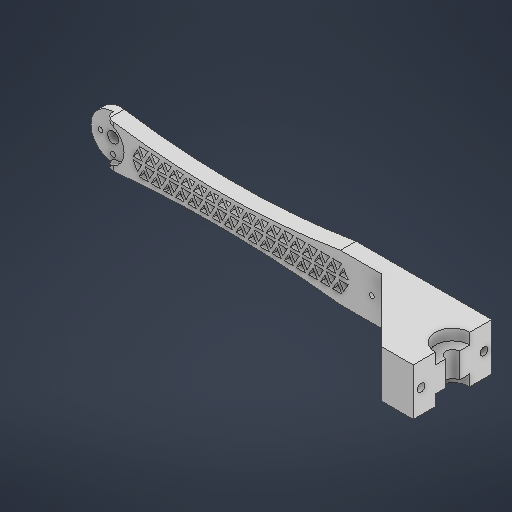
# Autodesk Inventor part: PeçaCerta
Saved by Autodesk Inventor 2026 (Build 300175050, 175E)
## iProperties
Created: 2025-03-07
Part Number: PeçaCerta
Material: Genérico
Document SubType Name: Modeling
Designer: Ian
Density: 1 g/cm^3
Appearance: Padrão
Mass: 116.041 g
Surface Area: 272.444 cm^2
Volume: 116.041 cm^3
Author: Ian
Autodesk Inventor part; units mm, degrees
ref_plane "YZ Plane" through (0, 0, 0) normal (1, 0, 0) x (0, 1, 0)
ref_plane "XZ Plane" through (0, 0, 0) normal (0, 1, 0) x (-1, 0, 0)
ref_plane "XY Plane" through (0, 0, 0) normal (0, 0, 1) x (1, 0, 0)
sketch "Esboço1" plane through (0, 0, 0) normal (0, 0, 1) x (1, 0, 0)
  circle A0 centre (-0.0013, -9.4999) radius 1.5997
  circle A1 centre (8, 0) radius 1.6001
  circle A2 centre (-8, 0) radius 1.5997
  circle A3 centre (0, 0) radius 3.5
  circle A4 centre (-0.0004, 9.5) radius 1.6001
  line L0 (0, 9.8096) -> (0, -11.1096)
  line L1 (-6.3022, 0) -> (16.3218, 0)
  line L2 (-14.0997, 15) -> (235.9003, 15)
  line L3 (235.9003, 15) -> (235.9003, -15)
  line L4 (235.9003, -15) -> (-14.0997, -15)
  line L5 (-14.0997, -15) -> (-14.0997, 15)
  point P0 (-14.0997, 0)
  dimension "d13" = 18.9999
  dimension "d37" = 9.2196
  dimension "d38" = 9.2197
  dimension "d39" = 9.2198
  dimension "d42" = 7
  dimension "d43" = 16
  dimension "d45" = 9.2207
  dimension "d46" = 4.5
  dimension "d47" = 250
  dimension "d48" = 30
  dimension "d49" = 0
  constraints: 12 end point, 5 centre point, 3 horizontal, 2 equal radius, 2 point on line, 2 vertical, 1 coincident, 1 midpoint, 1 parallel, 1 perpendicular
  measures "d13" distance of A4.centre A0.centre
  measures "d42" diameter of A3
  measures "d43" distance of A1.centre A2.centre
  measures "d46" distance edge to line of A2 L5
  measures "d47" distance of L2.start L2.end
  measures "d48" distance of L4.end L2.start
  measures "d49" vertical distance of A3.centre point (-14.1, 0)
extrude "Extrusão7" add sketch "Esboço1" along normal blind 10
sketch "Esboço13" plane through (0, 0, 0) normal (0, 0, -1) x (-1, 0, 0)
  line L0 (14.0997, -15) -> (-235.9003, -15) projected
  circle A0 centre (8, 0) radius 1.5997 projected
  circle A1 centre (0, 0) radius 3.5 projected
  circle A2 centre (0.0013, -9.4999) radius 1.5997 projected
  circle A3 centre (-8, 0) radius 1.6001 projected
  circle A4 centre (0.0004, 9.5) radius 1.6001 projected
  circle A5 centre (0, 0) radius 3.5
  circle A6 centre (-8, 0) radius 1.6001
  circle A7 centre (0.0013, -9.4999) radius 1.5997
  circle A8 centre (8, 0) radius 1.5997
  circle A9 centre (0.0004, 9.5) radius 1.6001
  line L1 (14.0997, 15) -> (14.0997, -15) projected
  line L2 (-14.0997, 15) -> (14.0997, 15)
  line L3 (14.0997, 15) -> (14.0997, -15)
  line L4 (14.0997, -15) -> (-14.0997, -15)
  line L5 (-14.0997, -15) -> (-14.0997, 15)
  line L6 (-14.0997, 15) -> (14.0997, -15) construction
  line L7 (14.0997, 15) -> (-14.0997, -15) construction
  circle A10 centre (0, 0) radius 14.0997
  point P0 (0, 0)
  point P1 (-15, -15)
  point P2 (-14.0997, -15)
  constraints: 12 end point, 6 centre point, 6 coincident, 5 concentric, 2 midpoint, 2 parallel, 1 horizontal, 1 perpendicular, 1 point on line
extrude "Extrusão11" add sketch "Esboço13" along normal blind 4
sketch "Esboço18" plane through (0, 0, 10) normal (0, 0, 1) x (1, 0, 0)
  line L0 (14.0997, -15) -> (235.9003, -15) projected
  line L1 (235.9003, 15) -> (14.0997, 15) projected
  line L2 (235.9003, -15) -> (175.9003, -15)
  line L3 (175.9003, -15) -> (175.9003, 15)
  line L4 (175.9003, 15) -> (235.9003, 15)
  line L5 (235.9003, 15) -> (235.9003, -15)
  point P0 (0, 0)
  dimension "d81" = 60
  constraints: 8 end point, 2 parallel, 1 horizontal, 1 perpendicular, 1 point on line
  measures "d81" distance of L3.end L4.end
extrude "Extrusão14" add sketch "Esboço18" along normal blind 40
sketch "Esboço19" plane through (14.0997, -15, 0) normal (0, -1, 0) x (1, 0, 0)
  line L0 (-28.1994, 10) -> (161.8006, 10) projected
  line L1 (161.8006, 10) -> (201.8006, 50)
  line L2 (221.8006, 50) -> (161.8006, 50) projected
  line L3 (201.8006, 50) -> (161.8006, 50)
  line L4 (161.8006, 10) -> (161.8006, 50)
  point P0 (-14.0997, 0)
  point P1 (0.4142, 10)
  point P2 (5, 10)
  point P3 (5, 10)
  point P4 (5.4142, 10)
  dimension "d84" = 45
  constraints: 6 end point, 1 collinear, 1 perpendicular, 1 point on line
  measures "d84" angle of L2 L1
extrude "Extrusão15" cut sketch "Esboço19" against normal through all
sketch "Esboço20" plane through (14.0997, -15, 0) normal (0, -1, 0) x (1, 0, 0)
  line L0 (161.8006, 10) -> (221.8006, 10)
  line L1 (221.8006, 0) -> (221.8006, 50) projected
  line L2 (221.8006, 50) -> (201.8006, 50) projected
  line L3 (201.8006, 50) -> (191.8006, 10)
  circle A0 centre (221.8006, 25) radius 10.975
  point P0 (-14.0997, 0)
  point P1 (221.8006, 35.975)
  point P2 (221.8006, 14.025)
  dimension "d87" = 21.95
  constraints: 4 end point, 2 midpoint, 1 centre point, 1 horizontal, 1 point on line
  measures "d87" diameter of A0
extrude "Extrusão16" cut sketch "Esboço20" against normal blind 7 contours A0 L1 picked at (218.1689, 24.559)
sketch "Esboço21" plane through (14.0997, -8, 0) normal (0, -1, 0) x (1, 0, 0)
  line L0 (221.8006, 35.975) -> (221.8006, 14.025) projected
  arc A0 (221.8006, 35.975) -> (221.8006, 14.025) centre (221.8006, 25) ccw projected
  circle A1 centre (221.8006, 25) radius 4.25
  point P0 (-14.0997, 0)
  point P1 (221.8006, 20.75)
  point P2 (221.8006, 29.25)
  dimension "d90" = 8.5
  constraints: 1 centre point, 1 coincident
  measures "d90" diameter of A1
extrude "Extrusão17" cut sketch "Esboço21" against normal through all contours L0 A1 picked at (220.3943, 24.8292)
sketch "Esboço22" plane through (14.0997, 15, 0) normal (0, 1, 0) x (1, 0, 0)
  arc A0 (221.8006, -20.75) -> (221.8006, -29.25) centre (221.8006, -25) ccw projected
  circle A1 centre (221.8006, -25) radius 10.975
  point P0 (-14.0997, 0)
  dimension "d93" = 21.95
  dimension "d173" = 4.25
  constraints: 1 centre point, 1 coincident
  measures "d93" diameter of A1
  measures "d173" radius of A0
extrude "Extrusão18" cut sketch "Esboço22" against normal blind 7
sketch "Esboço23" plane through (235.9003, -15, 0) normal (1, 0, 0) x (0, 0, -1)
  line L0 (-14.025, 30) -> (-14.025, 23) projected
  line L1 (-14.025, 7) -> (-14.025, 0) projected
  line L2 (-10, 0) -> (-10, 30) projected
  line L3 (-10, 30) -> (0, 30)
  circle A0 centre (-5, 15) radius 2.5
  line L4 (0, 15) -> (-50, 15)
  line L5 (-50, 30) -> (-50, 0) projected
  line L6 (-20.75, 23) -> (-20.75, 7) projected
  circle A1 centre (-45, 15) radius 2.5
  line L7 (-29.25, 7) -> (-29.25, 23) projected
  dimension "d96" = 5
  dimension "d174" = 15.75
  dimension "d175" = 5
  dimension "d177" = 15.75
  constraints: 4 end point, 2 centre point, 1 horizontal, 1 midpoint, 1 point on line
  measures "d96" diameter of A0
  measures "d174" distance from line of L6 A0.centre
  measures "d175" diameter of A1
  measures "d177" distance from line of L7 A1.centre
extrude "Extrusão19" cut sketch "Esboço23" against normal blind 50
sketch "Esboço24" plane through (0, 0, 0) normal (0, 0, -1) x (-1, 0, 0)
  line L0 (-235.9003, -2.5) -> (-235.9003, 2.5) projected
  line L1 (-175.9003, -15) -> (-175.9003, 15) projected
  line L2 (-183.4003, -12.5) -> (-208.4003, -12.5)
  line L3 (-208.4003, -12.5) -> (-208.4003, 12.5)
  line L4 (-208.4003, 12.5) -> (-183.4003, 12.5)
  line L5 (-183.4003, 12.5) -> (-183.4003, -12.5)
  line L6 (-183.4003, -12.5) -> (-208.4003, 12.5) construction
  line L7 (-208.4003, -12.5) -> (-183.4003, 12.5) construction
  point P0 (0, 0)
  dimension "d101" = 25
  dimension "d102" = 25
  constraints: 12 end point, 2 parallel, 1 horizontal, 1 perpendicular
  measures "d101" distance of L3.end L4.end
  measures "d102" distance of L2.end L3.end
extrude "Extrusão20" cut sketch "Esboço24" against normal through all
sketch "Esboço33" plane through (0, 0, 0) normal (0, 0, -1) x (-1, 0, 0)
  line L0 (-235.9003, -15) -> (-235.9003, 15) projected
  circle A0 centre (-169.6038, 0) radius 1.5
  point P0 (0, 0)
  dimension "d121" = 3
  dimension "d122" = 66.2965
  constraints: 1 centre point, 1 coincident
  measures "d121" diameter of A0
  measures "d122" distance from line of A0.centre L0
extrude "Extrusão25" cut sketch "Esboço33" against normal blind 10
sketch "Esboço42" plane through (0, 0, 50) normal (0, 0, 1) x (1, 0, 0)
  line L0 (208.4003, 12.5) -> (208.4003, 0) projected
  line L1 (208.4003, 0) -> (208.4003, -12.5) projected
  line L2 (215.9003, 15) -> (215.9003, -15) projected
  line L3 (208.4003, 12.5) -> (215.9003, 12.5)
  line L4 (215.9003, 12.5) -> (215.9003, -12.5)
  line L5 (215.9003, -12.5) -> (208.4003, -12.5)
  line L6 (208.4003, -12.5) -> (208.4003, 12.5)
  point P0 (0, 0)
  constraints: 8 end point, 2 parallel, 1 horizontal, 1 perpendicular, 1 point on line
extrude "Extrusão33" cut sketch "Esboço42" against normal blind 10
chamfer "Chanfro1" distance 7.5 angle 45 1 edges at (208.4003, 0, 40)
sketch "Esboço47" plane through (0, 0, -4) normal (0, 0, -1) x (-1, 0, 0)
  circle A0 centre (0, 0) radius 14.0997
  line L0 (-183.4003, -12.5) -> (-208.4003, -12.5) projected
  line L1 (-208.4003, -12.5) -> (-208.4003, 12.5) projected
  line L2 (-208.4003, 12.5) -> (-183.4003, 12.5) projected
  circle A1 centre (-169.6038, 0) radius 1.5 projected
  line L3 (-14.0997, -15) -> (-14.0997, 15) projected
  line L4 (-235.9003, 15) -> (-14.0997, 15) projected
  line L5 (-235.9003, -15) -> (-235.9003, 15) projected
  line L6 (-14.0997, -15) -> (-235.9003, -15) projected
  line L7 (-149.6038, 15) -> (-149.6038, -15)
  arc A2 (-149.6038, 15) -> (-2.1347, 13.9372) centre (-72.5593, 473.7324) ccw
  arc A3 (-1.4726, -14.0226) -> (-149.6038, -15) centre (-71.1626, -677.6545) ccw
  line L8 (-14.0997, -15) -> (14.0997, -15)
  line L9 (14.0997, -15) -> (14.0997, 15)
  line L10 (14.0997, 15) -> (-14.0997, 15)
  line L11 (-183.4003, 12.5) -> (-183.4003, -12.5) projected
  point P0 (14.0997, 0)
  dimension "d259" = 20
  dimension "d260" = 28.1994
  constraints: 8 end point, 6 point on circle, 3 centre point, 3 perpendicular, 2 point on line, 2 tangent, 1 coincident, 1 horizontal
  measures "d259" distance from line of A1.centre L7
  measures "d260" diameter of A0
extrude "Extrusão37" cut sketch "Esboço47" against normal through all contours L9 L8 L3 A3 A0 | A0 A2 L3 L10 L9 | A2 L4 L3 | L3 L6 A3
sketch "Esboço48" plane through (0, 0, 0) normal (0, 0, -1) x (-1, 0, 0)
  circle A0 centre (-169.6038, 0) radius 1.5 projected
  line L0 (-183.4003, -12.5) -> (-208.4003, -12.5) projected
  line L1 (-208.4003, -12.5) -> (-208.4003, 12.5) projected
  line L2 (-208.4003, 12.5) -> (-183.4003, 12.5) projected
  arc A1 (-14.0997, -12.8178) -> (-149.6038, -15) centre (-71.1626, -677.6545) ccw projected
  line L3 (-14.0997, -12.8178) -> (-14.0997, 12.2633) projected
  arc A2 (-149.6038, 15) -> (-14.0997, 12.2633) centre (-72.5593, 473.7324) ccw projected
  line L4 (-235.9003, 15) -> (-149.6038, 15) projected
  line L5 (-235.9003, -15) -> (-235.9003, 15) projected
  line L6 (-149.6038, -15) -> (-235.9003, -15) projected
  line L7 (-149.6038, 15) -> (-149.6038, -15)
  arc A3 (-14.0997, 12.2633) -> (-2.1347, 13.9372) centre (-72.5593, 473.7324) ccw projected
  line L8 (-14.0997, 12.2633) -> (-14.0997, -12.8178)
  line L9 (-147.6038, 12.2633) -> (-147.6038, -12.8178)
  arc A4 (-16.0997, -9.7446) -> (-147.6038, -12.8178) centre (-66.2789, -677.6545) ccw
  arc A5 (-147.6038, 12.2633) -> (-16.0997, 9.5965) centre (-72.5593, 469.1594) ccw
  line L10 (-16.0997, 9.5965) -> (-16.0997, -9.7446)
  line L11 (-147.6038, -0.2773) -> (-16.0997, -0.0741)
  line L12 (-140.8251, 0.7332) -> (-146.6038, 0.7243)
  line L13 (-146.6038, 0.7243) -> (-143.7222, 5.7332)
  line L14 (-143.7222, 5.7332) -> (-140.8251, 0.7332)
  line L15 (-136.0222, 5.7451) -> (-133.1251, 0.7451)
  line L16 (-138.9038, 0.7362) -> (-136.0222, 5.7451)
  line L17 (-133.1251, 0.7451) -> (-138.9038, 0.7362)
  line L18 (-128.3222, 5.757) -> (-125.4252, 0.757)
  line L19 (-131.2038, 0.7481) -> (-128.3222, 5.757)
  line L20 (-125.4252, 0.757) -> (-131.2038, 0.7481)
  line L21 (-120.6222, 5.7689) -> (-117.7252, 0.7689)
  line L22 (-123.5038, 0.76) -> (-120.6222, 5.7689)
  line L23 (-117.7252, 0.7689) -> (-123.5038, 0.76)
  line L24 (-112.9222, 5.7808) -> (-110.0252, 0.7808)
  line L25 (-115.8038, 0.7719) -> (-112.9222, 5.7808)
  line L26 (-110.0252, 0.7808) -> (-115.8038, 0.7719)
  line L27 (-105.2222, 5.7927) -> (-102.3252, 0.7927)
  line L28 (-108.1038, 0.7838) -> (-105.2222, 5.7927)
  line L29 (-102.3252, 0.7927) -> (-108.1038, 0.7838)
  line L30 (-97.5223, 5.8046) -> (-94.6252, 0.8046)
  line L31 (-100.4039, 0.7957) -> (-97.5223, 5.8046)
  line L32 (-94.6252, 0.8046) -> (-100.4039, 0.7957)
  line L33 (-89.8223, 5.8165) -> (-86.9252, 0.8165)
  line L34 (-92.7039, 0.8076) -> (-89.8223, 5.8165)
  line L35 (-86.9252, 0.8165) -> (-92.7039, 0.8076)
  line L36 (-82.1223, 5.8284) -> (-79.2252, 0.8284)
  line L37 (-85.0039, 0.8195) -> (-82.1223, 5.8284)
  line L38 (-79.2252, 0.8284) -> (-85.0039, 0.8195)
  line L39 (-74.4223, 5.8403) -> (-71.5252, 0.8403)
  line L40 (-77.3039, 0.8314) -> (-74.4223, 5.8403)
  line L41 (-71.5252, 0.8403) -> (-77.3039, 0.8314)
  line L42 (-66.7223, 5.8522) -> (-63.8252, 0.8522)
  line L43 (-69.6039, 0.8433) -> (-66.7223, 5.8522)
  line L44 (-63.8252, 0.8522) -> (-69.6039, 0.8433)
  line L45 (-59.0223, 5.8641) -> (-56.1252, 0.8641)
  line L46 (-61.9039, 0.8552) -> (-59.0223, 5.8641)
  line L47 (-56.1252, 0.8641) -> (-61.9039, 0.8552)
  line L48 (-51.3223, 5.876) -> (-48.4252, 0.876)
  line L49 (-54.2039, 0.8671) -> (-51.3223, 5.876)
  line L50 (-48.4252, 0.876) -> (-54.2039, 0.8671)
  line L51 (-43.6223, 5.8879) -> (-40.7253, 0.8879)
  line L52 (-46.5039, 0.879) -> (-43.6223, 5.8879)
  line L53 (-40.7253, 0.8879) -> (-46.5039, 0.879)
  line L54 (-35.9223, 5.8998) -> (-33.0253, 0.8998)
  line L55 (-38.8039, 0.8909) -> (-35.9223, 5.8998)
  line L56 (-33.0253, 0.8998) -> (-38.8039, 0.8909)
  line L57 (-28.2223, 5.9117) -> (-25.3253, 0.9117)
  line L58 (-31.1039, 0.9028) -> (-28.2223, 5.9117)
  line L59 (-25.3253, 0.9117) -> (-31.1039, 0.9028)
  line L60 (-20.5223, 5.9236) -> (-17.6253, 0.9236)
  line L61 (-23.4039, 0.9147) -> (-20.5223, 5.9236)
  line L62 (-17.6253, 0.9236) -> (-23.4039, 0.9147)
  line L63 (-139.8681, 3.0708) -> (-142.76, 8.0619)
  line L64 (-142.76, 8.0619) -> (-136.9916, 8.0708)
  line L65 (-136.9916, 8.0708) -> (-139.8681, 3.0708)
  line L66 (-132.1681, 3.0827) -> (-135.06, 8.0738)
  line L67 (-135.06, 8.0738) -> (-129.2916, 8.0827)
  line L68 (-129.2916, 8.0827) -> (-132.1681, 3.0827)
  line L69 (-124.4681, 3.0946) -> (-127.36, 8.0857)
  line L70 (-127.36, 8.0857) -> (-121.5916, 8.0946)
  line L71 (-121.5916, 8.0946) -> (-124.4681, 3.0946)
  line L72 (-116.7681, 3.1065) -> (-119.66, 8.0975)
  line L73 (-119.66, 8.0975) -> (-113.8917, 8.1065)
  line L74 (-113.8917, 8.1065) -> (-116.7681, 3.1065)
  line L75 (-109.0681, 3.1184) -> (-111.96, 8.1094)
  line L76 (-111.96, 8.1094) -> (-106.1917, 8.1184)
  line L77 (-106.1917, 8.1184) -> (-109.0681, 3.1184)
  line L78 (-101.3681, 3.1303) -> (-104.26, 8.1213)
  line L79 (-104.26, 8.1213) -> (-98.4917, 8.1303)
  line L80 (-98.4917, 8.1303) -> (-101.3681, 3.1303)
  line L81 (-93.6681, 3.1422) -> (-96.56, 8.1332)
  line L82 (-96.56, 8.1332) -> (-90.7917, 8.1422)
  line L83 (-90.7917, 8.1422) -> (-93.6681, 3.1422)
  line L84 (-85.9681, 3.1541) -> (-88.86, 8.1451)
  line L85 (-88.86, 8.1451) -> (-83.0917, 8.1541)
  line L86 (-83.0917, 8.1541) -> (-85.9681, 3.1541)
  line L87 (-78.2682, 3.166) -> (-81.1601, 8.157)
  line L88 (-81.1601, 8.157) -> (-75.3917, 8.166)
  line L89 (-75.3917, 8.166) -> (-78.2682, 3.166)
  line L90 (-70.5682, 3.1779) -> (-73.4601, 8.1689)
  line L91 (-73.4601, 8.1689) -> (-67.6917, 8.1779)
  line L92 (-67.6917, 8.1779) -> (-70.5682, 3.1779)
  line L93 (-62.8682, 3.1898) -> (-65.7601, 8.1808)
  line L94 (-65.7601, 8.1808) -> (-59.9917, 8.1898)
  line L95 (-59.9917, 8.1898) -> (-62.8682, 3.1898)
  line L96 (-55.1682, 3.2016) -> (-58.0601, 8.1927)
  line L97 (-58.0601, 8.1927) -> (-52.2917, 8.2016)
  line L98 (-52.2917, 8.2016) -> (-55.1682, 3.2016)
  line L99 (-47.4682, 3.2135) -> (-50.3601, 8.2046)
  line L100 (-50.3601, 8.2046) -> (-44.5917, 8.2135)
  line L101 (-44.5917, 8.2135) -> (-47.4682, 3.2135)
  line L102 (-39.7682, 3.2254) -> (-42.6601, 8.2165)
  line L103 (-42.6601, 8.2165) -> (-36.8917, 8.2254)
  line L104 (-36.8917, 8.2254) -> (-39.7682, 3.2254)
  line L105 (-32.0682, 3.2373) -> (-34.9601, 8.2284)
  line L106 (-34.9601, 8.2284) -> (-29.1918, 8.2373)
  line L107 (-29.1918, 8.2373) -> (-32.0682, 3.2373)
  line L108 (-24.3682, 3.2492) -> (-27.2601, 8.2403)
  line L109 (-27.2601, 8.2403) -> (-21.4918, 8.2492)
  line L110 (-21.4918, 8.2492) -> (-24.3682, 3.2492)
  line L111 (-140.822, -1.2668) -> (-146.6007, -1.2757)
  line L112 (-146.6007, -1.2757) -> (-143.7036, -6.2757)
  line L113 (-143.7036, -6.2757) -> (-140.822, -1.2668)
  line L114 (-136.0037, -6.2638) -> (-133.1221, -1.2549)
  line L115 (-138.9007, -1.2638) -> (-136.0037, -6.2638)
  line L116 (-133.1221, -1.2549) -> (-138.9007, -1.2638)
  line L117 (-128.3037, -6.2519) -> (-125.4221, -1.243)
  line L118 (-131.2007, -1.2519) -> (-128.3037, -6.2519)
  line L119 (-125.4221, -1.243) -> (-131.2007, -1.2519)
  line L120 (-120.6037, -6.24) -> (-117.7221, -1.2311)
  line L121 (-123.5007, -1.24) -> (-120.6037, -6.24)
  line L122 (-117.7221, -1.2311) -> (-123.5007, -1.24)
  line L123 (-112.9037, -6.2281) -> (-110.0221, -1.2192)
  line L124 (-115.8007, -1.2281) -> (-112.9037, -6.2281)
  line L125 (-110.0221, -1.2192) -> (-115.8007, -1.2281)
  line L126 (-105.2037, -6.2162) -> (-102.3221, -1.2073)
  line L127 (-108.1008, -1.2162) -> (-105.2037, -6.2162)
  line L128 (-102.3221, -1.2073) -> (-108.1008, -1.2162)
  line L129 (-97.5037, -6.2043) -> (-94.6221, -1.1954)
  line L130 (-100.4008, -1.2043) -> (-97.5037, -6.2043)
  line L131 (-94.6221, -1.1954) -> (-100.4008, -1.2043)
  line L132 (-89.8037, -6.1924) -> (-86.9221, -1.1835)
  line L133 (-92.7008, -1.1924) -> (-89.8037, -6.1924)
  line L134 (-86.9221, -1.1835) -> (-92.7008, -1.1924)
  line L135 (-82.1037, -6.1805) -> (-79.2221, -1.1716)
  line L136 (-85.0008, -1.1805) -> (-82.1037, -6.1805)
  line L137 (-79.2221, -1.1716) -> (-85.0008, -1.1805)
  line L138 (-74.4037, -6.1686) -> (-71.5221, -1.1597)
  line L139 (-77.3008, -1.1686) -> (-74.4037, -6.1686)
  line L140 (-71.5221, -1.1597) -> (-77.3008, -1.1686)
  line L141 (-66.7037, -6.1567) -> (-63.8221, -1.1478)
  line L142 (-69.6008, -1.1567) -> (-66.7037, -6.1567)
  line L143 (-63.8221, -1.1478) -> (-69.6008, -1.1567)
  line L144 (-59.0037, -6.1448) -> (-56.1221, -1.1359)
  line L145 (-61.9008, -1.1448) -> (-59.0037, -6.1448)
  line L146 (-56.1221, -1.1359) -> (-61.9008, -1.1448)
  line L147 (-51.3038, -6.1329) -> (-48.4222, -1.124)
  line L148 (-54.2008, -1.1329) -> (-51.3038, -6.1329)
  line L149 (-48.4222, -1.124) -> (-54.2008, -1.1329)
  line L150 (-43.6038, -6.121) -> (-40.7222, -1.1121)
  line L151 (-46.5008, -1.121) -> (-43.6038, -6.121)
  line L152 (-40.7222, -1.1121) -> (-46.5008, -1.121)
  line L153 (-35.9038, -6.1091) -> (-33.0222, -1.1002)
  line L154 (-38.8008, -1.1091) -> (-35.9038, -6.1091)
  line L155 (-33.0222, -1.1002) -> (-38.8008, -1.1091)
  line L156 (-28.2038, -6.0972) -> (-25.3222, -1.0883)
  line L157 (-31.1008, -1.0972) -> (-28.2038, -6.0972)
  line L158 (-25.3222, -1.0883) -> (-31.1008, -1.0972)
  line L159 (-20.5038, -6.0853) -> (-17.6222, -1.0764)
  line L160 (-23.4009, -1.0853) -> (-20.5038, -6.0853)
  line L161 (-17.6222, -1.0764) -> (-23.4009, -1.0853)
  line L162 (-139.8578, -3.6014) -> (-142.7342, -8.6014)
  line L163 (-142.7342, -8.6014) -> (-136.9659, -8.5925)
  line L164 (-136.9659, -8.5925) -> (-139.8578, -3.6014)
  line L165 (-132.1578, -3.5895) -> (-135.0342, -8.5895)
  line L166 (-135.0342, -8.5895) -> (-129.2659, -8.5806)
  line L167 (-129.2659, -8.5806) -> (-132.1578, -3.5895)
  line L168 (-124.4578, -3.5776) -> (-127.3342, -8.5776)
  line L169 (-127.3342, -8.5776) -> (-121.5659, -8.5687)
  line L170 (-121.5659, -8.5687) -> (-124.4578, -3.5776)
  line L171 (-116.7578, -3.5657) -> (-119.6343, -8.5657)
  line L172 (-119.6343, -8.5657) -> (-113.8659, -8.5568)
  line L173 (-113.8659, -8.5568) -> (-116.7578, -3.5657)
  line L174 (-109.0578, -3.5538) -> (-111.9343, -8.5538)
  line L175 (-111.9343, -8.5538) -> (-106.1659, -8.5449)
  line L176 (-106.1659, -8.5449) -> (-109.0578, -3.5538)
  line L177 (-101.3578, -3.5419) -> (-104.2343, -8.5419)
  line L178 (-104.2343, -8.5419) -> (-98.4659, -8.533)
  line L179 (-98.4659, -8.533) -> (-101.3578, -3.5419)
  line L180 (-93.6578, -3.53) -> (-96.5343, -8.53)
  line L181 (-96.5343, -8.53) -> (-90.7659, -8.5211)
  line L182 (-90.7659, -8.5211) -> (-93.6578, -3.53)
  line L183 (-85.9578, -3.5181) -> (-88.8343, -8.5181)
  line L184 (-88.8343, -8.5181) -> (-83.0659, -8.5092)
  line L185 (-83.0659, -8.5092) -> (-85.9578, -3.5181)
  line L186 (-78.2578, -3.5062) -> (-81.1343, -8.5062)
  line L187 (-81.1343, -8.5062) -> (-75.3659, -8.4973)
  line L188 (-75.3659, -8.4973) -> (-78.2578, -3.5062)
  line L189 (-70.5579, -3.4943) -> (-73.4343, -8.4943)
  line L190 (-73.4343, -8.4943) -> (-67.666, -8.4854)
  line L191 (-67.666, -8.4854) -> (-70.5579, -3.4943)
  line L192 (-62.8579, -3.4824) -> (-65.7343, -8.4824)
  line L193 (-65.7343, -8.4824) -> (-59.966, -8.4735)
  line L194 (-59.966, -8.4735) -> (-62.8579, -3.4824)
  line L195 (-55.1579, -3.4705) -> (-58.0343, -8.4705)
  line L196 (-58.0343, -8.4705) -> (-52.266, -8.4616)
  line L197 (-52.266, -8.4616) -> (-55.1579, -3.4705)
  line L198 (-47.4579, -3.4586) -> (-50.3343, -8.4586)
  line L199 (-50.3343, -8.4586) -> (-44.566, -8.4497)
  line L200 (-44.566, -8.4497) -> (-47.4579, -3.4586)
  line L201 (-39.7579, -3.4467) -> (-42.6344, -8.4467)
  line L202 (-42.6344, -8.4467) -> (-36.866, -8.4378)
  line L203 (-36.866, -8.4378) -> (-39.7579, -3.4467)
  line L204 (-32.0579, -3.4348) -> (-34.9344, -8.4348)
  line L205 (-34.9344, -8.4348) -> (-29.166, -8.4259)
  line L206 (-29.166, -8.4259) -> (-32.0579, -3.4348)
  line L207 (-24.3579, -3.4229) -> (-27.2344, -8.4229)
  line L208 (-27.2344, -8.4229) -> (-21.466, -8.414)
  line L209 (-21.466, -8.414) -> (-24.3579, -3.4229)
  line L210 (-144.6659, -8.6044) -> (-150.4445, -8.6133)
  line L211 (-150.4445, -8.6133) -> (-147.5629, -3.6044)
  line L212 (-147.5629, -3.6044) -> (-144.6659, -8.6044)
  line L213 (-144.6916, 8.0589) -> (-150.4703, 8.0499)
  line L214 (-150.4703, 8.0499) -> (-147.5732, 3.0499)
  line L215 (-147.5732, 3.0499) -> (-144.6916, 8.0589)
  line L216 (-154.5136, -1.6398) -> (-148.7349, -1.6309)
  line L217 (-148.7349, -1.6309) -> (-151.6165, -6.6398)
  line L218 (-151.6165, -6.6398) -> (-154.5136, -1.6398)
  line L219 (-148.7349, 1.0182) -> (-154.5228, 1.043)
  line L220 (-154.5228, 1.043) -> (-151.6073, 6.043)
  line L221 (-151.6073, 6.043) -> (-148.7349, 1.0182)
  line L222 (-183.4003, 12.5) -> (-183.4003, -12.5) projected
  point P0 (0, 0)
  point P1 (-143.717, 2.3969)
  point P2 (-136.0171, 2.4088)
  point P3 (-128.3171, 2.4207)
  point P4 (-120.6171, 2.4326)
  point P5 (-112.9171, 2.4445)
  point P6 (-105.2171, 2.4564)
  point P7 (-97.5171, 2.4683)
  point P8 (-89.8171, 2.4802)
  point P9 (-82.1171, 2.4921)
  point P10 (-74.4171, 2.504)
  point P11 (-66.7171, 2.5159)
  point P12 (-59.0171, 2.5278)
  point P13 (-51.3172, 2.5397)
  point P14 (-43.6172, 2.5516)
  point P15 (-35.9172, 2.5635)
  point P16 (-28.2172, 2.5754)
  point P17 (-20.5172, 2.5873)
  point P18 (-139.8732, 6.4011)
  point P19 (-138.4299, 5.5708)
  point P20 (-141.314, 5.5663)
  point P21 (-133.614, 5.5782)
  point P22 (-132.1732, 6.413)
  point P23 (-130.7299, 5.5827)
  point P24 (-125.914, 5.5901)
  point P25 (-124.4732, 6.4249)
  point P26 (-123.0299, 5.5946)
  point P27 (-118.2141, 5.602)
  point P28 (-116.7733, 6.4368)
  point P29 (-115.3299, 5.6065)
  point P30 (-110.5141, 5.6139)
  point P31 (-109.0733, 6.4487)
  point P32 (-107.6299, 5.6184)
  point P33 (-102.8141, 5.6258)
  point P34 (-101.3733, 6.4606)
  point P35 (-99.9299, 5.6303)
  point P36 (-95.1141, 5.6377)
  point P37 (-93.6733, 6.4725)
  point P38 (-92.2299, 5.6422)
  point P39 (-87.4141, 5.6496)
  point P40 (-85.9733, 6.4844)
  point P41 (-84.5299, 5.6541)
  point P42 (-79.7141, 5.6615)
  point P43 (-78.2733, 6.4963)
  point P44 (-76.8299, 5.666)
  point P45 (-72.0141, 5.6734)
  point P46 (-70.5733, 6.5082)
  point P47 (-69.1299, 5.6779)
  point P48 (-64.3141, 5.6853)
  point P49 (-62.8733, 6.5201)
  point P50 (-61.4299, 5.6898)
  point P51 (-56.6141, 5.6972)
  point P52 (-55.1733, 6.532)
  point P53 (-53.73, 5.7016)
  point P54 (-48.9141, 5.7091)
  point P55 (-47.4733, 6.5439)
  point P56 (-46.03, 5.7135)
  point P57 (-41.2142, 5.721)
  point P58 (-39.7733, 6.5558)
  point P59 (-38.33, 5.7254)
  point P60 (-33.5142, 5.7329)
  point P61 (-32.0734, 6.5677)
  point P62 (-30.63, 5.7373)
  point P63 (-25.8142, 5.7448)
  point P64 (-24.3734, 6.5796)
  point P65 (-22.93, 5.7492)
  point P66 (-16.0698, -9.7446)
  point P67 (-143.7088, -2.9394)
  point P68 (-136.0088, -2.9275)
  point P69 (-128.3088, -2.9156)
  point P70 (-120.6088, -2.9037)
  point P71 (-112.9088, -2.8918)
  point P72 (-105.2088, -2.8799)
  point P73 (-97.5089, -2.868)
  point P74 (-89.8089, -2.8561)
  point P75 (-82.1089, -2.8442)
  point P76 (-74.4089, -2.8323)
  point P77 (-66.7089, -2.8204)
  point P78 (-59.0089, -2.8085)
  point P79 (-51.3089, -2.7966)
  point P80 (-43.6089, -2.7847)
  point P81 (-35.9089, -2.7728)
  point P82 (-28.2089, -2.7609)
  point P83 (-20.5089, -2.749)
  point P84 (-139.8526, -6.9317)
  point P85 (-138.4118, -6.0969)
  point P86 (-141.296, -6.1014)
  point P87 (-133.596, -6.0895)
  point P88 (-132.1526, -6.9198)
  point P89 (-130.7118, -6.085)
  point P90 (-125.896, -6.0776)
  point P91 (-124.4526, -6.9079)
  point P92 (-123.0118, -6.0731)
  point P93 (-118.196, -6.0657)
  point P94 (-116.7527, -6.896)
  point P95 (-115.3119, -6.0612)
  point P96 (-110.496, -6.0538)
  point P97 (-109.0527, -6.8841)
  point P98 (-107.6119, -6.0493)
  point P99 (-102.796, -6.0419)
  point P100 (-101.3527, -6.8722)
  point P101 (-99.9119, -6.0374)
  point P102 (-95.0961, -6.03)
  point P103 (-93.6527, -6.8603)
  point P104 (-92.2119, -6.0255)
  point P105 (-87.3961, -6.0181)
  point P106 (-85.9527, -6.8484)
  point P107 (-84.5119, -6.0136)
  point P108 (-79.6961, -6.0062)
  point P109 (-78.2527, -6.8365)
  point P110 (-76.8119, -6.0017)
  point P111 (-71.9961, -5.9943)
  point P112 (-70.5527, -6.8247)
  point P113 (-69.1119, -5.9898)
  point P114 (-64.2961, -5.9824)
  point P115 (-62.8527, -6.8128)
  point P116 (-61.4119, -5.9779)
  point P117 (-56.5961, -5.9705)
  point P118 (-55.1527, -6.8009)
  point P119 (-53.7119, -5.966)
  point P120 (-48.8961, -5.9586)
  point P121 (-47.4527, -6.789)
  point P122 (-46.0119, -5.9541)
  point P123 (-41.1961, -5.9467)
  point P124 (-39.7527, -6.7771)
  point P125 (-38.3119, -5.9422)
  point P126 (-33.4961, -5.9348)
  point P127 (-32.0528, -6.7652)
  point P128 (-30.612, -5.9303)
  point P129 (-25.7961, -5.9229)
  point P130 (-24.3528, -6.7533)
  point P131 (-22.912, -5.9184)
  point P132 (-34.2417, 7.7295)
  point P133 (-34.6514, 7.6957)
  point P134 (-37.3181, 7.4844)
  point P135 (-42.0411, 7.1482)
  point P136 (-45.3226, 6.9431)
  point P137 (-49.4976, 6.716)
  point P138 (-57.7159, -7.9171)
  point P139 (-54.5451, -7.9651)
  point P140 (-53.2452, 6.5443)
  point P141 (-57.0225, 6.4021)
  point P142 (-61.0884, 6.2834)
  point P143 (-64.6178, 6.2094)
  point P144 (-60.3046, -7.889)
  point P145 (-65.3779, -7.8629)
  point P146 (-68.0256, -7.8646)
  point P147 (-73.0907, -7.897)
  point P148 (-68.8548, 6.1561)
  point P149 (-72.2853, 6.1414)
  point P150 (-84.1659, 6.2868)
  point P151 (-87.8452, 6.3937)
  point P152 (-76.5466, 6.1585)
  point P153 (-80.027, 6.2015)
  point P154 (-80.0823, -8.0046)
  point P155 (-75.6955, -7.9285)
  point P156 (-91.7147, 6.5377)
  point P157 (-95.7424, 6.7221)
  point P158 (-99.1948, 6.9081)
  point P159 (-103.721, 7.1911)
  point P160 (-106.6079, 7.3949)
  point P161 (-109.4506, 7.6133)
  point P162 (-29.2286, 8.1733)
  point P163 (-52.5314, -8.0034)
  point P164 (-80.8551, -8.0209)
  point P165 (-111.7841, 7.8058)
  point P166 (-113.9555, 7.9955)
  point P167 (-115.152, 8.1045)
  point P168 (-96.1652, -8.5294)
  point P169 (-90.8856, -8.3145)
  point P170 (-83.3152, -8.079)
  point P171 (-88.6725, -8.2368)
  point P172 (-44.7049, -8.2099)
  point P173 (-50.1037, -8.0577)
  point P174 (-42.5402, -8.2831)
  point P175 (-38.4606, -8.4402)
  point P176 (-147.5578, -6.9407)
  point P177 (-147.5784, 6.3862)
  point P178 (-151.6217, -3.3035)
  point P179 (-150.1757, -4.1353)
  point P180 (-151.6217, 2.7014)
  point P181 (-149.0217, 5.5499)
  point P182 (-149.6038, -7.1519)
  point P183 (-149.6038, -8.612)
  point P184 (-149.6038, -3.1412)
  point P185 (-149.6038, -1.6322)
  point P186 (-149.6038, 1.0219)
  point P187 (-149.6038, 2.5381)
  point P188 (-149.6038, 8.0513)
  point P189 (-149.6038, 6.5545)
  dimension "d263" = 2
  dimension "d264" = 2
  dimension "d265" = 0
  dimension "d266" = 0
  dimension "d268" = 2
  dimension "d269" = 5
  dimension "d270" = 1
  dimension "d273" = 7.7
  dimension "d279" = 2
  dimension "d280" = 2
  dimension "d283" = 7.7
  dimension "d291" = 1.9316
  dimension "d292" = 1.9316
  dimension "d293" = 5
  dimension "d295" = 5
  dimension "d296" = 2
  dimension "d299" = 2
  dimension "d300" = 5
  dimension "d301" = 0
  constraints: 430 end point, 169 symmetric about line, 6 midpoint, 3 parallel, 3 vertical, 2 point on circle, 1 centre point, 1 collinear, 289 other
  measures "d263" distance between parallel lines of L3 L10
  measures "d264" distance between parallel lines of L7 L9
  measures "d265" horizontal distance of A2.centre point (-72.559, 469.159)
  measures "d266" vertical distance of A1.centre A4.centre
  measures "d268" diameter of L12 L11
  measures "d269" vertical distance of L13.end L12.start
  measures "d270" distance from line of L9 L12.end
  measures "d273" distance of L12.start L15.end
  measures "d279" distance from line of L16 point (-138.43, 5.571)
  measures "d280" distance from line of L14 point (-141.314, 5.566)
  measures "d283" distance of L63.end L66.end
  measures "d291" distance of L162.end L210.start
  measures "d292" distance of L165.end L164.start
  measures "d293" vertical distance of L211.end L210.start
  measures "d295" vertical distance of L217.end L216.start
  measures "d296" distance from line of L211 point (-150.176, -4.135)
  measures "d299" distance from line of point (-149.022, 5.55) L221
  measures "d300" vertical distance of L219.end L220.end
  measures "d301" horizontal distance of L216.end L219.start
extrude "Extrusão38" cut sketch "Esboço48" against normal blind 50 contours L210 L211 L7 | L7 L211 L9 L210 | L9 L211 L212 L210 | L213 L9 L214 L7 | L7 L214 L213 | L217 L218 L216 L7 | L7 L216 L217 | L213 L215 L214 L9 | L181 L180 L182 A4 | L221 L219 L7 | L7 L219 L220 L221 | A5 L74 L72 L73 | L183 L185 A4 | L107 L105 A5 | A4 L201 L203 L202 | A5 L77 L75 | L186 L188 A4 | L104 L102 A5 | A4 L198 L200 | A5 L80 L78 | L189 L191 A4 | L101 L99 A5 | A4 L195 L197 | A5 L83 L81 | L192 L194 A4 | L98 L96 A5 | A5 L86 L84 | L95 L93 A5 | A5 L89 L87 | L92 L90 A5 | L12 L13 L14 | L15 L17 L16 | L18 L20 L19 | L21 L23 L22 | L24 L26 L25 | L27 L29 L28 | L30 L32 L31 | L33 L35 L34 | L36 L38 L37 | L39 L41 L40 | L42 L44 L43 | L45 L47 L46 | L48 L50 L49 | L51 L53 L52 | L54 L56 L55 | L57 L59 L58 | L60 L62 L61 | L63 L64 L65 | L66 L67 L68 | L69 L70 L71 | L108 L109 L110 | L113 L112 L111 | L115 L116 L114 | L118 L119 L117 | L121 L122 L120 | L124 L125 L123 | L127 L128 L126 | L130 L131 L129 | L133 L134 L132 | L136 L137 L135 | L139 L140 L138 | L142 L143 L141 | L145 L146 L144 | L148 L149 L147 | L151 L152 L150 | L154 L155 L153 | L157 L158 L156 | L160 L161 L159 | L164 L163 L162 | L167 L166 L165 | L170 L169 L168 | L173 L172 L171 | L176 L175 L174 | L179 L178 L177 | L206 L205 L204 | L209 L208 L207
sketch "Esboço49" plane through (0, 0, 10) normal (0, 0, 1) x (1, 0, 0)
  circle A0 centre (0, 0) radius 12
  arc A1 (0, 14.0997) -> (0, -14.0997) centre (0, 0) ccw
  line L0 (0, -14.0997) -> (0, -12)
  line L1 (0, 12) -> (0, 14.0997)
  dimension "d304" = 24
  constraints: 4 end point, 4 point on circle, 2 centre point, 2 coincident, 2 vertical
  measures "d304" diameter of A0
extrude "Extrusão39" cut sketch "Esboço49" against normal blind 5
fillet "Arredondamento9" radius 5 2 edges at (0, -13.0499, 10) (0, 13.0499, 10)
sketch "Esboço50" plane through (0, 0, -4) normal (0, 0, -1) x (-1, 0, 0)
  circle A0 centre (0.0004, 9.5) radius 1.6001 projected
  circle A1 centre (-8, 0) radius 1.6001 projected
  circle A2 centre (0.0013, -9.4999) radius 1.5997 projected
  circle A3 centre (0, 0) radius 3.5 projected
  circle A4 centre (8, 0) radius 1.5997 projected
  arc A5 (-1.4726, -14.0226) -> (-14.0997, -12.8178) centre (-71.1626, -677.6545) ccw projected
  arc A6 (-1.4726, -14.0226) -> (-2.1347, 13.9372) centre (0, 0) ccw projected
  arc A7 (-14.0997, 12.2633) -> (-2.1347, 13.9372) centre (-72.5593, 473.7324) ccw projected
  line L0 (-14.0997, 12.2633) -> (-14.0997, -12.8178) projected
extrude "Extrusão40" cut sketch "Esboço50" against normal up to surface (4 mm away)
fillet "Arredondamento10" radius 2 4 edges at (183.4003, 12.5, 8.75) (208.4003, 12.5, 16.2501) (208.4003, -12.5, 16.2501) (183.4003, -12.5, 8.75)
